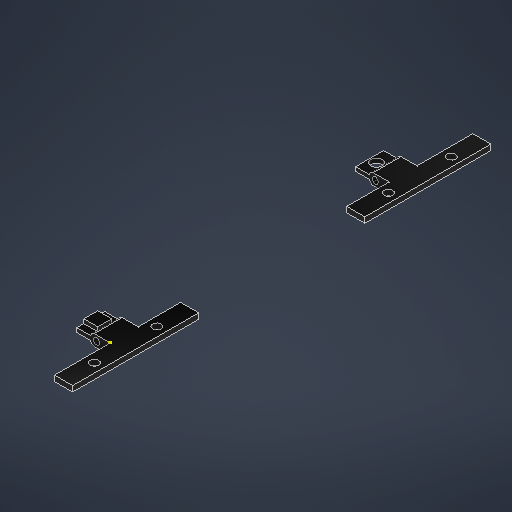
# Autodesk Inventor part: mocowanie do pługu
Saved by Autodesk Inventor 2026.2 (Build 302298010, 298A)
## iProperties
Created: 2026-05-09
Part Number: mocowanie do pługu
Material: Tworzywo sztuczne PET
Document SubType Name: Modeling
Designer: karol
Density: 1.541 g/cm^3
Appearance: Poliwęglan — przezroczysty
Author: karol
Autodesk Inventor part; units mm, degrees
ref_plane "YZ Plane" through (0, 0, 0) normal (1, 0, 0) x (0, 1, 0)
ref_plane "XZ Plane" through (0, 0, 0) normal (0, 1, 0) x (-1, 0, 0)
ref_plane "XY Plane" through (0, 0, 0) normal (0, 0, 1) x (1, 0, 0)
sketch "Sketch21" plane through (0, 0, 0) normal (0, 1, 0) x (-1, 0, 0)
  line L0 (0, 0) -> (7, 0)
  line L1 (7, 0) -> (7, -10)
  line L2 (7, -10) -> (0, -10)
  line L3 (0, -10) -> (0, 0)
  line L4 (0, -100) -> (7, -100)
  line L5 (7, -100) -> (7, -110)
  line L6 (7, -110) -> (0, -110)
  line L7 (0, -110) -> (0, -100)
  dimension "d144" = 7
  dimension "d145" = 10
  dimension "d146" = 7
  dimension "d147" = 10
  dimension "d148" = 90
  constraints: 16 end point, 4 parallel, 2 horizontal, 2 perpendicular, 1 collinear
  measures "d144" distance of L1.end L2.end
  measures "d145" distance of L0.end L1.end
  measures "d146" distance of L5.end L6.end
  measures "d147" distance of L4.end L5.end
  measures "d148" distance between parallel lines of L2 L4
extrude "Extrusion19" add sketch "Sketch21" along normal blind 4
sketch "Sketch22" plane through (0, 0, 0) normal (1, 0, 0) x (0, 0, -1)
  line L0 (10, 4) -> (0, 4) projected
  line L1 (10, 0) -> (10, 4) projected
  line L2 (0, 4) -> (10, 4)
  line L3 (10, 4) -> (10, 2)
  line L4 (10, 2) -> (0, 2)
  line L5 (0, 2) -> (0, 4)
  line L6 (10, 4) -> (25.2, 4)
  line L7 (25.2, 4) -> (25.2, 2)
  line L8 (25.2, 2) -> (10, 2)
  line L9 (10, 2) -> (10, 4)
  line L10 (0, 4) -> (-20, 4)
  line L11 (-20, 4) -> (-20, 2)
  line L12 (-20, 2) -> (0, 2)
  line L13 (0, 2) -> (0, 4)
  line L14 (110, 0) -> (110, 4) projected
  line L15 (100, 4) -> (110, 4)
  line L16 (110, 4) -> (110, 2)
  line L17 (110, 2) -> (100, 2)
  line L18 (100, 2) -> (100, 4)
  line L19 (100, 2) -> (84.8, 2)
  line L20 (84.8, 2) -> (84.8, 4)
  line L21 (84.8, 4) -> (100, 4)
  line L22 (100, 4) -> (100, 2)
  line L23 (110, 4) -> (130, 4)
  line L24 (130, 4) -> (130, 2)
  line L25 (130, 2) -> (110, 2)
  line L26 (110, 2) -> (110, 4)
  point P0 (0, 0)
  point P1 (10, 3)
  point P2 (0, 3)
  dimension "d151" = 10
  dimension "d152" = 15.2
  dimension "d153" = 20
  dimension "d154" = 15.2
  dimension "d155" = 20
  constraints: 48 end point, 12 parallel, 6 horizontal, 6 perpendicular, 4 midpoint, 2 point on line
  measures "d151" distance of point (10, 3) point (0, 3)
  measures "d152" distance of L7.end L8.end
  measures "d153" distance of L12.end L11.end
  measures "d154" distance of L20.end L21.end
  measures "d155" distance of L24.end L25.end
extrude "Extrusion20" add sketch "Sketch22" along normal blind 6.5
sketch "Sketch23" plane through (0, 4, 0) normal (0, 1, 0) x (1, 0, 0)
  point P0 (0, 0)
sketch "Sketch24" plane through (0, 4, 0) normal (0, 1, 0) x (1, 0, 0)
  circle A0 centre (3.25, -9) radius 1.55
  circle A1 centre (3.25, 13.5) radius 1.55
  line L0 (0, -20) -> (6.5, -20) projected
  line L1 (0, 0) -> (0, -20) projected
  line L2 (0, 25.2) -> (0, 10) projected
  circle A2 centre (3.25, 96.5) radius 1.55
  circle A3 centre (3.25, 119) radius 1.55
  line L3 (0, 130) -> (0, 110) projected
  line L4 (0, 130) -> (6.5, 130) projected
  point P0 (3.25, -20)
  point P1 (3.25, -20)
  point P2 (3.25, 130)
  point P3 (3.25, 130)
  dimension "d158" = 3.1
  dimension "d159" = 3.1
  dimension "d160" = 11
  dimension "d161" = 33.5
  dimension "d162" = 3.25
  dimension "d163" = 3.25
  dimension "d164" = 3.1
  dimension "d165" = 3.1
  dimension "d166" = 3.25
  dimension "d167" = 11
  dimension "d169" = 33.5
  dimension "d170" = 3.25
  constraints: 4 centre point, 4 midpoint
  measures "d158" diameter of A0
  measures "d159" diameter of A1
  measures "d160" distance of point (3.25, -20) A0.centre
  measures "d161" distance of point (3.25, -20) A1.centre
  measures "d162" distance from line of L1 A0.centre
  measures "d163" distance from line of L2 A1.centre
  measures "d164" diameter of A2
  measures "d165" diameter of A3
  measures "d166" distance from line of L3 A3.centre
  measures "d167" distance of point (3.25, 130) A3.centre
  measures "d169" distance of point (3.25, 130) A2.centre
  measures "d170" distance from line of L3 A2.centre
extrude "Extrusion21" cut sketch "Sketch24" against normal blind 2
sketch "Sketch25" plane through (-7, 0, 0) normal (0, 0, 1) x (1, 0, 0)
  circle A0 centre (2, 2) radius 1.15
  line L0 (0, 0) -> (0, 4) projected
  line L1 (0, 4) -> (7, 4) projected
  point P0 (7, 0)
  point P1 (0, 2)
  dimension "d173" = 2.3
  dimension "d174" = 2
  dimension "d175" = 2
  constraints: 1 centre point, 1 midpoint
  measures "d173" diameter of A0
  measures "d174" distance of point (0, 2) A0.centre
  measures "d175" distance from line of L1 A0.centre
extrude "Extrusion22" cut sketch "Sketch25" against normal blind 90
fillet "Fillet5" radius 1.25 4 edges at (-7, 0, -5) (-7, 4, -5) (-7, 0, -105) (-7, 4, -105)
sketch "Szkic26" plane through (0, 0, -100) normal (0, 0, 1) x (1, 0, 0)
  line L0 (0, 2) -> (6.5, 2) projected
  circle A0 centre (-5, 2) radius 1.15 projected
  point P0 (0, 0)
extrude "Wyciągnięcie proste23" cut sketch "Szkic26" against normal blind 10
sketch "Sketch27" plane through (-7, 1.25, -110) normal (-1, 0, 0) x (0, 0, 1)
  line L0 (110, 0) -> (100, 0) projected
  line L1 (100, 1.5) -> (110, 1.5) projected
  line L2 (100, 0) -> (110, 0)
  line L3 (110, 0) -> (110, 1.5)
  line L4 (110, 1.5) -> (100, 1.5)
  line L5 (100, 1.5) -> (100, 0)
  line L6 (0, -1.25) -> (0, 0.75) projected
  line L7 (10, 1.9) -> (10, -0.4) projected
  line L8 (0, 0) -> (10, 0)
  line L9 (10, 0) -> (10, 1.5)
  line L10 (10, 1.5) -> (0, 1.5)
  line L11 (0, 1.5) -> (0, 0)
  point P0 (110, -1.25)
  constraints: 16 end point, 4 parallel, 4 point on line, 2 horizontal, 2 perpendicular
extrude "Extrusion24" add sketch "Sketch27" along normal blind 5
sketch "Szkic28" plane through (-12, 1.25, 0) normal (0, -1, 0) x (1, 0, 0)
  circle A0 centre (2.5, -5) radius 2
  line L0 (5, -10) -> (0, -10) projected
  line L1 (0, -10) -> (0, 0) projected
  circle A1 centre (2.5, -105) radius 2
  line L2 (5, -110) -> (0, -110) projected
  line L3 (0, -110) -> (0, -100) projected
  point P0 (12, 0)
  point P1 (0, -5)
  point P2 (2.5, -110)
  dimension "d183" = 4
  dimension "d184" = 5
  dimension "d185" = 2.5
  dimension "d186" = 4
  dimension "d187" = 5
  dimension "d188" = 2.5
  constraints: 2 centre point, 2 midpoint
  measures "d183" diameter of A0
  measures "d184" distance from line of L0 A0.centre
  measures "d185" distance of point (0, -5) A0.centre
  measures "d186" diameter of A1
  measures "d187" distance of point (2.5, -110) A1.centre
  measures "d188" distance from line of L3 A1.centre
extrude "Wyciągnięcie proste25" cut sketch "Szkic28" against normal blind 2
sketch "Szkic29" plane through (-12, 2.75, -110) normal (0, 1, 0) x (1, 0, 0)
  circle A0 centre (2.5, -105) radius 2 projected
  circle A1 centre (2.5, -105) radius 2
  circle A2 centre (2.5, -5) radius 2 projected
  circle A3 centre (2.5, -5) radius 2
  line L0 (0, -110) -> (0, -100) projected
  line L1 (0, -107.5) -> (5, -107.5)
  line L2 (5, -107.5) -> (5, -102.5)
  line L3 (5, -102.5) -> (0, -102.5)
  line L4 (0, -102.5) -> (0, -107.5)
  line L5 (5, -100) -> (0, -100) projected
  point P0 (12, -110)
  point P1 (0, -102.5)
  dimension "d191" = 5
  dimension "d192" = 5
  dimension "d193" = 2.5
  constraints: 8 end point, 2 centre point, 2 coincident, 2 parallel, 1 horizontal, 1 perpendicular, 1 point on line
  measures "d191" distance of L3.end L2.end
  measures "d192" distance of L2.end L1.end
  measures "d193" distance between parallel lines of L5 L3
extrude "Wyciągnięcie proste26" add sketch "Szkic29" along normal blind 1.5 contours L0 L3 L2 L1
sketch "Szkic30" plane through (-12, 4.25, -110) normal (0, 1, 0) x (1, 0, 0)
  circle A0 centre (2.5, -105) radius 2 projected
  circle A1 centre (2.5, -105) radius 2
  point P0 (12, -110)
  constraints: 1 centre point, 1 coincident
extrude "Wyciągnięcie proste27" add sketch "Szkic30" against normal blind 0.5
body "Solid2"
